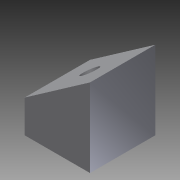
# Autodesk Inventor part: hack 35 degree mounting points
Saved by Autodesk Inventor 2011 SP1 (Build 150282100, 282)
## iProperties
Created: 2013-01-18
Part Number: hack 35 degree mounting points
Document SubType Name: Modeling
Designer: wes
Density: 1 g/cm^3
Author: wes
Autodesk Inventor part; units mm, degrees
ref_plane "YZ Plane" through (0, 0, 0) normal (1, 0, 0) x (0, 1, 0)
ref_plane "XZ Plane" through (0, 0, 0) normal (0, 1, 0) x (-1, 0, 0)
ref_plane "XY Plane" through (0, 0, 0) normal (0, 0, 1) x (1, 0, 0)
sketch "Sketch1" plane through (0, 0, 0) normal (0, 0, 1) x (1, 0, 0)
  line L0 (-16.2275, -3.6228) -> (9.1725, 14.1625)
  line L1 (9.1725, 14.1625) -> (9.1725, -16.3228)
  line L2 (9.1725, -16.3228) -> (-16.2275, -16.3228)
  line L3 (-16.2275, -16.3228) -> (-16.2275, -3.6228)
  dimension "d6" = 35
  dimension "d7" = 12.7
  dimension "d8" = 25.4
  constraints: 8 end point, 2 perpendicular, 1 vertical
  measures "d6" angle of L2 L0
  measures "d7" distance of L2.end L0.start
  measures "d8" distance of L1.end L2.end
extrude "Extrusion1" add sketch "Sketch1" along normal blind 25.4
sketch "Sketch2" plane through (9.1725, 14.1625, 25.4) normal (-0.5736, 0.8192, 0) x (0.8192, 0.5736, 0)
  circle A0 centre (-15.6369, 12.7) radius 3.175
  point P0 (-15.6369, 25.4)
  dimension "d11" = 6.35
  constraints: 1 centre point
  measures "d11" diameter of A0
extrude "Extrusion2" cut sketch "Sketch2" against normal blind 12.7
sketch "Sketch3" plane through (-16.2275, -16.3228, 0) normal (0, -1, 0) x (1, 0, 0)
  circle A0 centre (12.7, 12.7) radius 3.175
  point P0 (16.2275, 0)
  dimension "d14" = 6.35
  constraints: 1 centre point
  measures "d14" diameter of A0
extrude "Extrusion3" cut sketch "Sketch3" against normal blind 10.16
body "Solid1"
